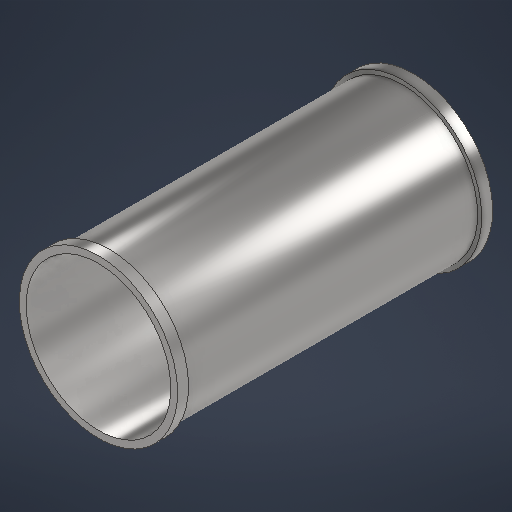
# Autodesk Inventor part: DiscoCorpoTurbina3
Saved by Autodesk Inventor 2026.2 (Build 302298010, 298A)
## iProperties
Created: 2026-04-30
Part Number: DiscoCorpoTurbina3
Material: Steel, Alloy
Document SubType Name: Modeling
Designer: Yan
Density: 7.73 g/cm^3
Appearance: Semi-Polished
Author: Yan
Autodesk Inventor part; units mm, degrees
ref_plane "YZ Plane" through (0, 0, 0) normal (1, 0, 0) x (0, 1, 0)
ref_plane "XZ Plane" through (0, 0, 0) normal (0, 1, 0) x (-1, 0, 0)
ref_plane "XY Plane" through (0, 0, 0) normal (0, 0, 1) x (1, 0, 0)
sketch "Sketch1" plane through (0, 0, 0) normal (1, 0, 0) x (0, 1, 0)
  line L0 (0, 0) -> (0, -1154)
  line L1 (0, -1154) -> (265, -1154)
  line L2 (265, -1154) -> (265, 0)
  line L3 (265, 0) -> (0, 0)
  line L4 (265, 0) -> (290, 0)
  line L5 (290, 0) -> (290, -40)
  line L6 (290, -40) -> (275, -40)
  line L7 (275, -40) -> (275, -1114)
  line L8 (275, -1114) -> (290, -1114)
  line L9 (290, -1114) -> (290, -1154)
  line L10 (265, -1154) -> (290, -1154)
  dimension "d16" = 530
  dimension "d17" = 550
  dimension "d18" = 580
  dimension "d19" = 40
  dimension "d20" = 40
  dimension "d21" = 1154
  constraints: 22 end point, 8 perpendicular, 4 point on line, 1 vertical
  measures "d16" diameter of L2 L0
  measures "d17" diameter of L7 L0
  measures "d18" diameter of L5 L0
  measures "d19" distance between parallel lines of L10 L8
  measures "d20" distance between parallel lines of L4 L6
  measures "d21" distance of L0.start L0.end
revolve "Revolution1" add sketch "Sketch1" angle 360 about axis through (0, 0, 0) along (0, 0, -1) contours L4 L5 L6 L7 L8 L9 L10 L2
body "Solid1"
